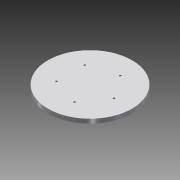
# Autodesk Inventor part: Hotplate Top 01
Saved by Autodesk Inventor 2015 (Build 190159000, 159)
## iProperties
Created: 2016-08-07
Part Number: Hotplate Top 01
Material: Generic
Document SubType Name: Modeling
Designer: spichelh
Density: 1 g/cm^3
Appearance: Default
Author: spichelh
Autodesk Inventor part; units mm, degrees
ref_plane "YZ Plane" through (0, 0, 0) normal (1, 0, 0) x (0, 1, 0)
ref_plane "XZ Plane" through (0, 0, 0) normal (0, 1, 0) x (-1, 0, 0)
ref_plane "XY Plane" through (0, 0, 0) normal (0, 0, 1) x (1, 0, 0)
sketch "Sketch1" plane through (0, 0, 0) normal (0, 1, 0) x (-1, 0, 0)
  circle A0 centre (0, 0) radius 70
  dimension "d0" = 140
  constraints: 1 centre point, 1 coincident
  measures "d0" diameter of A0
extrude "Extrusion1" add sketch "Sketch1" along normal blind 7
sketch "Sketch2" plane through (0, 0, 0) normal (0, -1, 0) x (1, 0, 0)
  circle A0 centre (0, 0) radius 62
  circle A1 centre (0, 0) radius 70 projected
  dimension "d3" = 8
  constraints: 1 centre point, 1 coincident
  measures "d3" radial gap between concentric circles of A0 A1
extrude "Extrusion2" cut sketch "Sketch2" against normal blind 4 contours A0
sketch "Sketch7" plane through (0, 4, 0) normal (0, -1, 0) x (1, 0, 0)
  line L0 (-55, -12.5) -> (-20, -12.5)
  line L1 (-18, -10.5) -> (-18, 10.5)
  line L2 (-20, 12.5) -> (-55, 12.5)
  line L3 (-57, 10.5) -> (-57, -10.5)
  line L4 (0, 0) -> (-42.9306, 0) construction
  arc A0 (-57, -10.5) -> (-55, -12.5) centre (-55, -10.5) ccw
  arc A1 (-55, 12.5) -> (-57, 10.5) centre (-55, 10.5) ccw
  arc A2 (-18, 10.5) -> (-20, 12.5) centre (-20, 10.5) ccw
  arc A3 (-20, -12.5) -> (-18, -10.5) centre (-20, -10.5) ccw
  line L5 (-5.1077, -56.1708) -> (5.7079, -22.8838)
  line L6 (4.4238, -20.3637) -> (-15.5484, -13.8743)
  line L7 (-18.0685, -15.1584) -> (-28.8841, -48.4454)
  line L8 (-27.6001, -50.9655) -> (-7.6279, -57.4549)
  arc A4 (-7.6279, -57.4549) -> (-5.1077, -56.1708) centre (-7.0098, -55.5528) ccw
  arc A5 (-28.8841, -48.4454) -> (-27.6001, -50.9655) centre (-26.982, -49.0634) ccw
  arc A6 (-15.5484, -13.8743) -> (-18.0685, -15.1584) centre (-16.1664, -15.7765) ccw
  arc A7 (5.7079, -22.8838) -> (4.4238, -20.3637) centre (3.8058, -22.2658) ccw
  line L9 (51.8433, -22.2155) -> (23.5277, -1.643)
  line L10 (20.7341, -2.0855) -> (8.3906, -19.0748)
  line L11 (8.833, -21.8684) -> (37.1486, -42.4409)
  line L12 (39.9422, -41.9984) -> (52.2857, -25.0091)
  arc A8 (52.2857, -25.0091) -> (51.8433, -22.2155) centre (50.6677, -23.8335) ccw
  arc A9 (37.1486, -42.4409) -> (39.9422, -41.9984) centre (38.3242, -40.8229) ccw
  arc A10 (8.3906, -19.0748) -> (8.833, -21.8684) centre (10.0086, -20.2504) ccw
  arc A11 (23.5277, -1.643) -> (20.7341, -2.0855) centre (22.3521, -3.261) ccw
  line L13 (37.1486, 42.4409) -> (8.833, 21.8684)
  line L14 (8.3906, 19.0748) -> (20.7341, 2.0855)
  line L15 (23.5277, 1.643) -> (51.8433, 22.2155)
  line L16 (52.2857, 25.0091) -> (39.9422, 41.9984)
  arc A12 (39.9422, 41.9984) -> (37.1486, 42.4409) centre (38.3242, 40.8229) ccw
  arc A13 (51.8433, 22.2155) -> (52.2857, 25.0091) centre (50.6677, 23.8335) ccw
  arc A14 (20.7341, 2.0855) -> (23.5277, 1.643) centre (22.3521, 3.261) ccw
  arc A15 (8.833, 21.8684) -> (8.3906, 19.0748) centre (10.0086, 20.2504) ccw
  line L17 (-28.8841, 48.4454) -> (-18.0685, 15.1584)
  line L18 (-15.5484, 13.8743) -> (4.4238, 20.3637)
  line L19 (5.7079, 22.8838) -> (-5.1077, 56.1708)
  line L20 (-7.6279, 57.4549) -> (-27.6001, 50.9655)
  arc A16 (-27.6001, 50.9655) -> (-28.8841, 48.4454) centre (-26.982, 49.0634) ccw
  arc A17 (-5.1077, 56.1708) -> (-7.6279, 57.4549) centre (-7.0098, 55.5528) ccw
  arc A18 (4.4238, 20.3637) -> (5.7079, 22.8838) centre (3.8058, 22.2658) ccw
  arc A19 (-18.0685, 15.1584) -> (-15.5484, 13.8743) centre (-16.1664, 15.7765) ccw
  point P0 (-18, 12.5)
  point P1 (-18, -12.5)
  point P2 (-57, 12.5)
  point P3 (-57, 0)
  point P4 (-17.4505, -13.2563)
  point P5 (6.3259, -20.9817)
  point P6 (-29.5022, -50.3475)
  point P7 (-17.614, -54.2102)
  point P8 (-13.2663, -40.8295)
  point P9 (7.215, -20.6928)
  point P10 (21.9096, -0.4674)
  point P11 (38.7667, -43.6165)
  point P12 (46.114, -33.5038)
  point P13 (34.7316, -25.234)
  point P14 (21.9096, 0.4674)
  point P15 (7.215, 20.6928)
  point P16 (53.4613, 23.391)
  point P17 (46.114, 33.5038)
  point P18 (34.7316, 25.234)
  point P19 (6.3259, 20.9817)
  point P20 (-17.4505, 13.2563)
  point P21 (-5.7258, 58.0729)
  point P22 (-17.614, 54.2102)
  point P23 (-13.2663, 40.8295)
  dimension "d35" = 25
  dimension "d36" = 39
  dimension "d37" = 18
  dimension "d38" = 2
  dimension "d41" = 360
  constraints: 42 end point, 40 point on circle, 31 point on line, 20 centre point, 8 tangent, 3 equal radius, 2 horizontal, 2 parallel, 1 midpoint, 1 perpendicular, 126 other
  measures "d35" distance of point (-18, -12.5) point (-18, 12.5)
  measures "d36" distance of point (-18, 12.5) point (-57, 12.5)
  measures "d37" distance from line of L4.start L1
  measures "d38" radius of A0
extrude "Extrusion5" cut sketch "Sketch7" against normal blind 2
sketch "Sketch8" plane through (0, 4, 0) normal (0, -1, 0) x (1, 0, 0)
  line L0 (24.1459, -1.1756) -> (8.5795, -22.6008)
  line L1 (6.3435, -23.3274) -> (-18.8435, -15.1437)
  line L2 (-20.2254, -13.2415) -> (-20.2254, 13.2415)
  line L3 (-18.8435, 15.1437) -> (6.3435, 23.3274)
  line L4 (8.5795, 22.6008) -> (24.1459, 1.1756)
  line L5 (0, 0) -> (38.0077, 0) construction
  arc A0 (24.1459, -1.1756) -> (24.1459, 1.1756) centre (22.5279, 0) ccw
  arc A1 (8.5795, 22.6008) -> (6.3435, 23.3274) centre (6.9615, 21.4253) ccw
  arc A2 (-18.8435, 15.1437) -> (-20.2254, 13.2415) centre (-18.2254, 13.2415) ccw
  arc A3 (-20.2254, -13.2415) -> (-18.8435, -15.1437) centre (-18.2254, -13.2415) ccw
  arc A4 (6.3435, -23.3274) -> (8.5795, -22.6008) centre (6.9615, -21.4253) ccw
  point P0 (25, 0)
  point P1 (7.7254, -23.7764)
  point P2 (-20.2254, -14.6946)
  point P3 (-20.2254, 14.6946)
  point P4 (7.7254, 23.7764)
  dimension "d48" = 25
  dimension "d49" = 2
  constraints: 12 end point, 11 point on line, 10 point on circle, 10 tangent, 5 centre point, 4 equal radius, 1 coincident, 1 horizontal, 11 other
  measures "d48" distance of point (0, 0) point (25, 0)
  measures "d49" radius of A0
extrude "Extrusion6" cut sketch "Sketch8" against normal blind 2
sketch "Sketch9" plane through (0, 0, 0) normal (0, -1, 0) x (1, 0, 0)
  circle A0 centre (0, 0) radius 67
  circle A1 centre (0, 0) radius 64
  circle A2 centre (0, 0) radius 62 projected
  dimension "d50" = 3
  dimension "d51" = 2
  constraints: 2 centre point, 2 coincident
  measures "d50" radial gap between concentric circles of A0 A1
  measures "d51" radial gap between concentric circles of A1 A2
extrude "Extrusion7" cut sketch "Sketch9" against normal blind 1.5 contours A0
fillet "Fillet1" radius 1.5 2 edges at (-67, 1.5, 0) (-64, 1.5, 0)
sketch "Sketch11" plane through (0, 0, 0) normal (0, -1, 0) x (1, 0, 0)
  line L0 (0, 0) -> (-70, 0) construction
  circle A0 centre (0, 0) radius 70 construction
  line L1 (0, 0) -> (-70, 0) construction
  line L2 (0, 0) -> (-69.7336, 6.1009) construction
  circle A1 centre (0, 0) radius 64 projected
  arc A2 (-63.7565, 5.578) -> (-64, 0) centre (0, 0) ccw
  arc A3 (-63.7565, 5.578) -> (-64, 0) centre (0, 0) ccw
  circle A4 centre (0, 0) radius 64 projected
  line L3 (-64, 0) -> (-64, 0)
  line L4 (-63.7565, 5.578) -> (-63.7565, 5.578)
  arc A5 (-69.7336, 6.1009) -> (-70, 0) centre (0, 0) ccw
  line L5 (-63.7565, 5.578) -> (-69.7336, 6.1009)
  line L6 (-64, 0) -> (-70, 0)
  dimension "d58" = 5
  constraints: 14 end point, 9 point on circle, 4 point on line, 3 centre point, 3 coincident, 3 collinear, 2 horizontal alignment, 1 horizontal, 2 other
  measures "d58" angle of L2 L0
sketch "Sketch13" plane through (0, 4, 0) normal (0, -1, 0) x (1, 0, 0)
  circle A0 centre (40, 0) radius 1.5
  line L0 (0, 0) -> (58.1181, 0) construction
  circle A1 centre (12.3607, 38.0423) radius 1.5
  line L1 (0, 0) -> (17.9595, 55.2736) construction
  circle A2 centre (-32.3607, 23.5114) radius 1.5
  line L2 (0, 0) -> (-47.0185, 34.1609) construction
  circle A3 centre (-32.3607, -23.5114) radius 1.5
  line L3 (0, 0) -> (-47.0185, -34.1609) construction
  circle A4 centre (12.3607, -38.0423) radius 1.5
  line L4 (0, 0) -> (17.9595, -55.2736) construction
  dimension "d65" = 3
  dimension "d66" = 40
  dimension "d71" = 360
  constraints: 10 end point, 5 centre point, 5 point on line, 2 coincident, 1 horizontal, 24 other
  measures "d65" diameter of A0
  measures "d66" distance of A0.centre L0.start
extrude "Extrusion9" cut sketch "Sketch13" against normal blind 4
sketch "Sketch14" plane through (0, 6, 0) normal (0, -1, 0) x (1, 0, 0)
  circle A0 centre (0, 0) radius 4
  dimension "d73" = 8
  constraints: 1 centre point, 1 coincident
  measures "d73" diameter of A0
extrude "Extrusion10" add sketch "Sketch14" along normal blind 15
body "Solid1"
